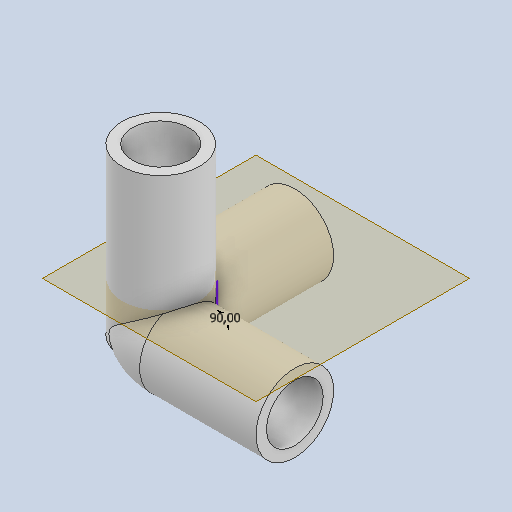
# Autodesk Inventor part: Knee-big-UP
Saved by Autodesk Inventor 2025 (Build 290162000, 162)
## iProperties
Created: 2025-09-15
Part Number: Knee-big-UP
Material: Generic
Document SubType Name: Modeling
Designer: Pravoslav
Density: 1 g/cm^3
Appearance: Default
Author: Pravoslav
Autodesk Inventor part; units mm, degrees
ref_plane "YZ Plane" through (0, 0, 0) normal (1, 0, 0) x (0, 1, 0)
ref_plane "XY Plane" through (0, 0, 0) normal (0, 0, 1) x (1, 0, 0)
sketch "Sketch1" plane through (0, 0, 0) normal (0, 0, 1) x (1, 0, 0)
  circle A0 centre (0, 0) radius 3.615
  circle A1 centre (0, 0) radius 5
  dimension "d0" = 7.23
  dimension "d1" = 10
  constraints: 2 centre point, 2 coincident
  measures "d0" diameter of A0
  measures "d1" diameter of A1
sketch "Sketch2" plane through (0, 0, 0) normal (0, 0, 1) x (1, 0, 0)
  line L0 (5.0177, 0) -> (5.0177, 4.7273)
  line L1 (5.0177, 0) -> (9.745, 0) construction
  line L2 (5.0177, 4.7273) -> (5.0177, -3.9213)
  point P0 (0, 0)
  dimension "d2" = 90
  constraints: 6 end point, 1 horizontal, 1 perpendicular, 1 point on line
  measures "d2" angle of L1 L0
revolve "Revolution1" add sketch "Sketch1" angle 90 about axis through (5.0177, 0, 0) along (0, 1, 0)
sketch "Sketch3" plane through (5.0177, 0, 5.0177) normal (1, 0, 0) x (0, 0, -1)
  point P0 (5.0177, 0)
sketch "Sketch4" plane through (5.0177, 0, 5.0177) normal (1, 0, 0) x (0, 0, -1)
  circle A0 centre (0, 0) radius 3.615
  circle A1 centre (0, 0) radius 5
  point P0 (5.0177, 0)
  dimension "d4" = 7.23
  dimension "d5" = 10
  constraints: 2 centre point, 1 coincident
  measures "d4" diameter of A0
  measures "d5" diameter of A1
extrude "Extrusion1" add sketch "Sketch4" along normal blind 15
sketch "Sketch5" plane through (0, 0, 0) normal (0, 0, -1) x (-1, 0, 0)
  circle A0 centre (0, 0) radius 3.615
  circle A1 centre (0, 0) radius 5
  dimension "d8" = 7.23
  dimension "d9" = 10
  constraints: 2 centre point, 2 coincident
  measures "d8" diameter of A0
  measures "d9" diameter of A1
extrude "Extrusion2" add sketch "Sketch5" along normal blind 15
ref_plane "Work Plane1" through (0, 5, 0) normal (0, 1, 0) x (-1, 0, 0)
sketch "Sketch6" plane through (0, 5, 0) normal (0, 1, 0) x (-1, 0, 0)
  circle A0 centre (-1.3677, 3.65) radius 5
  circle A1 centre (-1.3677, 3.65) radius 3.65
  line L0 (-5.0177, 10.0177) -> (-5.0177, 0.0177) projected
  point P0 (0, 0)
  dimension "d12" = 10
  dimension "d13" = 7.3
  dimension "d15" = 3.65
  dimension "d16" = 3.65
  constraints: 2 centre point, 1 coincident
  measures "d12" diameter of A0
  measures "d13" diameter of A1
  measures "d15" vertical distance of A0.centre point (0, 0)
  measures "d16" distance from line of L0 A0.centre
extrude "Extrusion3" add sketch "Sketch6" along normal blind 15 and the other way blind 6.25
sketch "Sketch7" plane through (1.3677, 20, 3.65) normal (0, 1, 0) x (1, 0, 0)
  circle A0 centre (0, 0) radius 3.65
  point P0 (-1.3677, 3.65)
  dimension "d21" = 7.3
  constraints: 1 centre point
  measures "d21" diameter of A0
extrude "Extrusion4" cut sketch "Sketch7" against normal blind 19.404
sketch "Sketch8" plane through (0, 0, -15) normal (0, 0, -1) x (-1, 0, 0)
  circle A0 centre (0, 0) radius 3.65
  dimension "d24" = 7.3
  constraints: 1 centre point, 1 coincident
  measures "d24" diameter of A0
extrude "Extrusion5" cut sketch "Sketch8" against normal blind 19.404
sketch "Sketch9" plane through (20.0177, 0, 5.0177) normal (1, 0, 0) x (0, 0, -1)
  circle A0 centre (0, 0) radius 3.65
  point P0 (5.0177, 0)
  dimension "d27" = 7.3
  constraints: 1 centre point
  measures "d27" diameter of A0
extrude "Extrusion6" cut sketch "Sketch9" against normal blind 19.404
body "Solid1"
